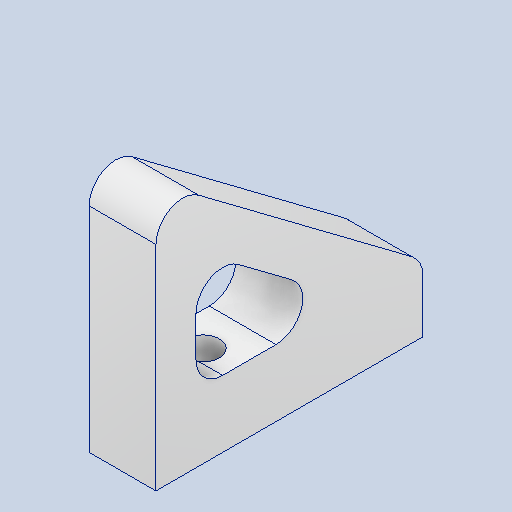
# Autodesk Inventor part: belt_liner_v5_Plate_11
Saved by Autodesk Inventor 2025.2 (Build 292293000, 293)
## iProperties
Created: 2025-02-23
Part Number: belt_liner_v5_Plate_11
Material: アルミニウム 6061
Document SubType Name: Modeling
Designer: haruy
Density: 2.7 g/cm^3
Appearance: アルミニウム - フラット
Author: haruy
Autodesk Inventor part; units mm, degrees
ref_plane "YZ Plane" through (0, 0, 0) normal (1, 0, 0) x (0, 1, 0)
ref_plane "XZ Plane" through (0, 0, 0) normal (0, 1, 0) x (-1, 0, 0)
ref_plane "XY Plane" through (0, 0, 0) normal (0, 0, 1) x (1, 0, 0)
sketch "スケッチ1" plane through (0, 0, 0) normal (1, 0, 0) x (0, 1, 0)
  line L0 (0, 0) -> (5, 0)
  line L1 (5, 0) -> (5, -20)
  line L2 (5, -20) -> (0, -20)
  line L3 (0, -20) -> (0, 0)
  line L4 (5, 0) -> (20, 0)
  line L5 (20, 0) -> (5, -20)
  line L6 (5, -3) -> (14, -3)
  line L7 (14, -3) -> (2.6, -18.2)
  point P0 (5, -15)
  dimension "d0" = 5
  dimension "d1" = 20
  dimension "d3" = 15
  dimension "d4" = 3
  constraints: 16 end point, 2 horizontal, 2 parallel, 1 perpendicular, 1 other
  measures "d0" distance of L1.end L2.end
  measures "d1" distance between parallel lines of L0 L2
  measures "d3" distance of L0.end L4.end
  measures "d4" distance between parallel lines of L4 L6
extrude "押し出し1" add sketch "スケッチ1" against normal blind 5 contours L0 L1 L2 L3 | L4 L5 L1 L7 L6
fillet "フィレット1" radius 2 5 edges at (-2.5, 20, 0) (-2.5, 5, -20) (-2.5, 5, -15) (-2.5, 5, -3) (-2.5, 14, -3)
sketch "スケッチ2" plane through (0, 0, -20) normal (0, -1, 0) x (1, 0, 0)
  line L0 (-5, 20) -> (0, 20) projected
  line L1 (-2.5, 20) -> (-2.5, 0)
  line L2 (0, 0) -> (-5, 0) projected
  point P0 (-2.5, 14)
  point P1 (-2.5, 7)
  dimension "d0" = 5
  dimension "d8" = 7
  dimension "d9" = 7
  constraints: 2 end point, 2 midpoint, 2 point on line
  measures "d8" distance of point (-2.5, 14) point (-2.5, 7)
  measures "d9" distance from line of L2 point (-2.5, 7)
hole "穴1" at (-2.5, 0, -6) at (-2.5, 0, -13) direction (0, 1, 0) diameter 2.5 depth 5 tip angle 118
